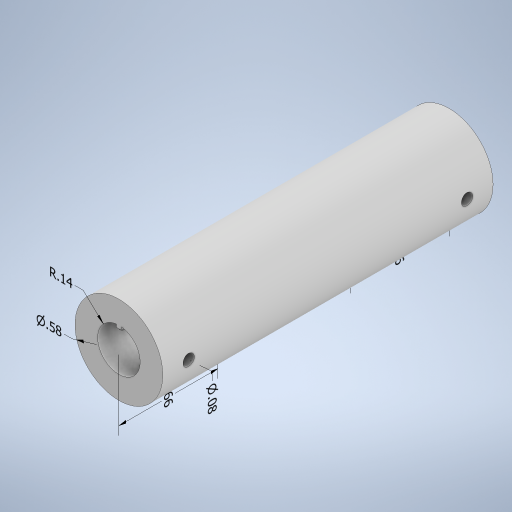
# Autodesk Inventor part: Wheel_axis
Saved by Autodesk Inventor 2023 (Build 270158000, 158)
## iProperties
Created: 2022-10-19
Part Number: Wheel_axis
Material: Generic
Document SubType Name: Modeling
Designer: guill
Density: 1 g/cm^3
Appearance: Default
Author: guill
## iProperties of the stored document Wheel_axis_3DPrint.ipt
Created: 2022-10-20
Part Number: Wheel_axis_3DPrint
Material: Generic
Document SubType Name: Modeling
Designer: guill
Density: 1 g/cm^3
Appearance: Default
Author: guill
Autodesk Inventor part; units mm, degrees
ref_plane "YZ Plane" through (0, 0, 0) normal (1, 0, 0) x (0, 1, 0)
ref_plane "XZ Plane" through (0, 0, 0) normal (0, 1, 0) x (-1, 0, 0)
ref_plane "XY Plane" through (0, 0, 0) normal (0, 0, 1) x (1, 0, 0)
sketch "Sketch1" plane through (0, 0, 0) normal (0, 0, 1) x (1, 0, 0)
  circle A0 centre (0, 0) radius 7.3825
  dimension "d0" = 14.765
  constraints: 1 centre point, 1 coincident
  measures "d0" diameter of A0
extrude "Extrusion1" add sketch "Sketch1" along normal mid plane 55.56
sketch "Sketch3" plane through (0, 0, 27.78) normal (0, 0, 1) x (1, 0, 0)
  circle A0 centre (0, 0) radius 3.5725
  dimension "d6" = 7.145
  constraints: 1 centre point, 1 coincident
  measures "d6" diameter of A0
extrude "Extrusion2" cut sketch "Sketch3" against normal blind 16.6675
sketch "Sketch4" plane through (0, 0, 0) normal (1, 0, 0) x (0, 1, 0)
  circle A0 centre (0, -23.4163) radius 0.9525
  point P0 (0, 0)
  dimension "d9" = 23.4163
  dimension "d10" = 1.905
  constraints: 1 centre point
  measures "d9" distance of point (0, 0) A0.centre
  measures "d10" diameter of A0
extrude "Extrusion3" cut sketch "Sketch4" along normal through all both and the other way through all
sketch "Sketch6" plane through (0, 0, 0) normal (1, 0, 0) x (0, 1, 0)
  line L0 (-3.5725, 27.78) -> (3.5725, 27.78) projected
  line L1 (-3.5725, 11.1125) -> (3.5725, 11.1125) projected
  line L2 (3.5725, 27.78) -> (3.0645, 27.78)
  line L3 (3.0645, 27.78) -> (3.0645, 11.1125)
  line L4 (3.0645, 11.1125) -> (3.5725, 11.1125)
  line L5 (3.5725, 11.1125) -> (3.5725, 27.78)
  point P0 (0, 0)
  dimension "d17" = 0.508
  constraints: 8 end point, 2 parallel, 1 horizontal, 1 perpendicular, 1 point on line
  measures "d17" distance of L2.end L0.end
extrude "Extrusion5" add sketch "Sketch6" along normal mid plane 0.8636
mirror "Mirror5" about plane through (0, 0, 0) normal (0, 0, 1) of "Extrusion5", "Extrusion3", "Extrusion2"
body "Solid1"
